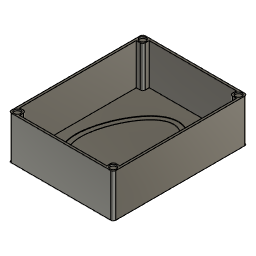
Wingspan - Eggs Container (Autodesk Fusion 360 design; units mm, degrees)
Autodesk Fusion 360 part; units mm, degrees
sketch "Skizze1" plane through (0, 0, 0) normal (0, 0, 1) x (1, 0, 0)
  line L0 (0, 0) -> (85, 0)
  line L1 (85, 0) -> (85, 109)
  line L2 (85, 109) -> (0, 109)
  line L3 (0, 109) -> (0, 0)
  dimension "d1" = 85
  dimension "d2" = 109
  constraint horizontal L0
  constraint vertical L1
  constraint horizontal L2
  constraint vertical L3
  constraint coincident L0.start L3.end
  measures "d1" distance of L0.start L0.end
  measures "d2" distance of L0.start L2.end
extrude "Extrusion16" add sketch "Skizze1" along normal blind 35
sketch "Skizze17" plane through (0, 0, 35) normal (0, 0, 1) x (-1, 0, 0)
  line L0 (0, -109) -> (0, 0)
  line L1 (0, 0) -> (-85, 0)
  line L2 (-85, 0) -> (-85, -109)
  line L3 (-85, -109) -> (0, -109)
  line L4 (0, -109) -> (-7, -109)
  line L5 (-7, -109) -> (-7, -102)
  line L6 (-7, -102) -> (0, -102)
  line L7 (0, -102) -> (0, -109)
  line L8 (-85, -109) -> (-78, -109)
  line L9 (-78, -109) -> (-78, -102)
  line L10 (-78, -102) -> (-85, -102)
  line L11 (-85, -102) -> (-85, -109)
  line L12 (0, 0) -> (-7, 0)
  line L13 (-7, 0) -> (-7, -7)
  line L14 (-7, -7) -> (0, -7)
  line L15 (0, -7) -> (0, 0)
  line L16 (-85, 0) -> (-78, 0)
  line L17 (-78, 0) -> (-78, -7)
  line L18 (-78, -7) -> (-85, -7)
  line L19 (-85, -7) -> (-85, 0)
  circle A0 centre (-3.5, -105.5) radius 2.65
  circle A1 centre (-81.5, -105.5) radius 2.65
  circle A2 centre (-81.5, -3.5) radius 2.65
  circle A3 centre (-3.5, -3.5) radius 2.65
  dimension "d148" = 7
  dimension "d149" = 7
  dimension "d150" = 7
  dimension "d151" = 7
  dimension "d152" = 7
  dimension "d153" = 7
  dimension "d154" = 7
  dimension "d155" = 7
  dimension "d156" = 5.3
  dimension "d157" = 5.3
  dimension "d158" = 5.3
  dimension "d159" = 5.3
  dimension "d160" = 3.5
  dimension "d161" = 3.5
  dimension "d162" = 3.5
  dimension "d163" = 3.5
  dimension "d164" = 3.5
  dimension "d165" = 3.5
  dimension "d166" = 3.5
  dimension "d167" = 3.5
  constraint horizontal L4
  constraint vertical L5
  constraint horizontal L6
  constraint vertical L7
  constraint coincident L0.start L3.end
  constraint horizontal L8
  constraint vertical L9
  constraint horizontal L10
  constraint vertical L11
  constraint coincident L2.end L3.start
  constraint horizontal L12
  constraint vertical L13
  constraint horizontal L14
  constraint vertical L15
  constraint coincident L0.end L1.start
  constraint horizontal L16
  constraint vertical L17
  constraint horizontal L18
  constraint vertical L19
  constraint coincident L1.end L2.start
  measures "d148" distance of L0.start L4.end
  measures "d149" distance of L0.start L6.end
  measures "d150" distance of L2.end L8.end
  measures "d151" distance of L2.end L10.end
  measures "d152" distance of L0.end L12.end
  measures "d153" distance of L0.end L14.end
  measures "d154" distance of L1.end L16.end
  measures "d155" distance of L1.end L18.end
  measures "d156" diameter of A0
  measures "d157" diameter of A1
  measures "d158" diameter of A2
  measures "d159" diameter of A3
  measures "d160" distance of L15 A3.centre
  measures "d161" distance of L14 A3.centre
  measures "d162" distance of L16 A2.centre
  measures "d163" distance of L19 A2.centre
  measures "d164" distance of L8 A1.centre
  measures "d165" distance of L11 A1.centre
  measures "d166" distance of L7 A0.centre
  measures "d167" distance of L4 A0.centre
sketch "Skizze18" plane through (0, 0, 35) normal (0, 0, 1) x (-1, 0, 0)
  line L0 (-78, -1.75) -> (-7, -1.75)
  line L1 (-7, -1.75) -> (-7, -107.25)
  line L2 (-7, -107.25) -> (-78, -107.25)
  line L3 (-78, -107.25) -> (-78, -1.75)
  line L4 (0, -109) -> (0, 0)
  line L5 (-78, 0) -> (-78, -7)
  line L6 (-85, 0) -> (-85, -109)
  line L7 (0, 0) -> (-85, 0)
  line L8 (-85, -109) -> (0, -109)
  dimension "d168" = 7
  dimension "d170" = 7
  dimension "d171" = 1.75
  dimension "d172" = 1.75
  constraint horizontal L0
  constraint vertical L1
  constraint horizontal L2
  constraint vertical L3
  measures "d168" distance of L1 L4
  measures "d170" distance of L3 L6
  measures "d171" distance of L0 L7
  measures "d172" distance of L2 L8
sketch "Skizze19" plane through (0, 0, 35) normal (0, 0, 1) x (-1, 0, 0)
  line L0 (-7, -7) -> (-1.75, -7)
  line L1 (-1.75, -7) -> (-1.75, -102)
  line L2 (-1.75, -102) -> (-7, -102)
  line L3 (-7, -102) -> (-7, -7)
  line L4 (0, 0) -> (-7, 0)
  line L5 (0, -109) -> (-7, -109)
  line L6 (0, -109) -> (0, 0)
  line L7 (-78, -7) -> (-83.25, -7)
  line L8 (-83.25, -7) -> (-83.25, -102)
  line L9 (-83.25, -102) -> (-78, -102)
  line L10 (-78, -102) -> (-78, -7)
  line L11 (-85, 0) -> (-85, -109)
  line L12 (-85, -109) -> (-78, -109)
  line L13 (-85, 0) -> (-78, 0)
  dimension "d174" = 7
  dimension "d175" = 7
  dimension "d176" = 7
  dimension "d177" = 1.75
  dimension "d178" = 1.75
  dimension "d179" = 7
  dimension "d180" = 7
  dimension "d181" = 7
  constraint horizontal L0
  constraint vertical L1
  constraint horizontal L2
  constraint vertical L3
  constraint horizontal L7
  constraint vertical L8
  constraint horizontal L9
  constraint vertical L10
  measures "d174" distance of L0 L4
  measures "d175" distance of L2 L5
  measures "d176" distance of L3 L6
  measures "d177" distance of L1 L6
  measures "d178" distance of L8 L11
  measures "d179" distance of L9 L12
  measures "d180" distance of L10 L11
  measures "d181" distance of L7 L13
extrude "Extrusion17" cut sketch "Skizze17" against normal blind 1.2 contours A0 | A1 | A2 | A3
extrude "Extrusion18" cut sketch "Skizze18" sketch "Skizze19" against normal blind 33.25 contours L0 L1 L2 L3 L5 of sketch 2
fillet "Abrundung5" radius 2 8 edges at (7, 102, 18.375) (78, 102, 18.375) (78, 7, 18.375) (7, 7, 18.375) (85, 109, 17.5) (0, 109, 17.5) (0, 0, 17.5) (85, 0, 17.5)
sketch "Skizze20" plane through (0, 0, 1.75) normal (0, 0, 1) x (-1, 0, 0)
  line L0 (-78, -104) -> (-78, -107.25)
  line L1 (-78, -107.25) -> (-7, -107.25)
  line L2 (-7, -107.25) -> (-7, -104)
  arc A0 (-5, -102) -> (-7, -104) centre (-5, -104) ccw
  line L3 (-5, -102) -> (-1.75, -102)
  line L4 (-1.75, -102) -> (-1.75, -7)
  line L5 (-1.75, -7) -> (-5, -7)
  arc A1 (-7, -5) -> (-5, -7) centre (-5, -5) ccw
  line L6 (-7, -5) -> (-7, -1.75)
  line L7 (-7, -1.75) -> (-78, -1.75)
  line L8 (-78, -1.75) -> (-78, -5)
  arc A2 (-80, -7) -> (-78, -5) centre (-80, -5) ccw
  line L9 (-80, -7) -> (-83.25, -7)
  line L10 (-83.25, -7) -> (-83.25, -102)
  line L11 (-83.25, -102) -> (-80, -102)
  arc A3 (-78, -104) -> (-80, -102) centre (-80, -104) ccw
  spline S0 degree 3 poles (-66.1211, -76.6115) (-59.4052, -88.6986) (-51.0157, -95.3555) (-42.4975, -95.3555) knots 0 0 0 0 1 1 1 1
  spline S1 degree 3 poles (-42.4975, -95.3555) (-33.9794, -95.3555) (-25.5902, -88.6986) (-18.874, -76.6115) knots 0 0 0 0 1 1 1 1
  spline S2 degree 3 poles (-18.874, -76.6115) (-13.324, -66.622) (-9.7378, -54.1768) (-9.7378, -44.9054) knots 0 0 0 0 1 1 1 1
  spline S3 degree 3 poles (-9.7378, -44.9054) (-9.7378, -35.9571) (-13.092, -27.5787) (-19.183, -21.3143) knots 0 0 0 0 1 1 1 1
  spline S4 degree 3 poles (-19.183, -21.3143) (-25.3273, -14.9941) (-33.6072, -11.5139) (-42.4979, -11.5139) knots 0 0 0 0 1 1 1 1
  spline S5 degree 3 poles (-42.4979, -11.5139) (-51.3886, -11.5139) (-59.6684, -14.9944) (-65.8128, -21.3143) knots 0 0 0 0 1 1 1 1
  spline S6 degree 3 poles (-65.8128, -21.3143) (-71.9035, -27.5791) (-75.2576, -35.9571) (-75.2576, -44.9054) knots 0 0 0 0 1 1 1 1
  spline S7 degree 3 poles (-75.2576, -44.9054) (-75.2573, -54.1768) (-71.671, -66.6223) (-66.1211, -76.6115) knots 0 0 0 0 1 1 1 1
  spline S8 degree 3 poles (-42.4975, -15.4416) (-26.3299, -15.4416) (-13.6658, -28.3836) (-13.6658, -44.9054) knots 0 0 0 0 1 1 1 1
  spline S9 degree 3 poles (-13.6658, -44.9054) (-13.6658, -62.4321) (-27.1411, -91.4275) (-42.4975, -91.4275) knots 0 0 0 0 1 1 1 1
  spline S10 degree 3 poles (-42.4975, -91.4275) (-57.854, -91.4275) (-71.3293, -62.4321) (-71.3293, -44.9054) knots 0 0 0 0 1 1 1 1
  spline S11 degree 3 poles (-71.3293, -44.9054) (-71.3293, -28.3836) (-58.6652, -15.4416) (-42.4975, -15.4416) knots 0 0 0 0 1 1 1 1
extrude "Extrusion19" cut sketch "Skizze20" against normal blind 0.4 contours S0 S1 S2 S3 S4 S5 S6 S7
extrude "Extrusion9" [suppressed]
sketch "Skizze14" plane through (0, 0, 35) normal (0, 0, 1) x (-1, 0, 0)
  line L0 (0, -115) -> (0, 0)
  line L1 (0, 0) -> (-85, 0)
  line L2 (-85, 0) -> (-85, -115)
  line L3 (-85, -115) -> (0, -115)
  line L4 (0, -115) -> (-7, -115)
  line L5 (-7, -115) -> (-7, -108)
  line L6 (-7, -108) -> (0, -108)
  line L7 (0, -108) -> (0, -115)
  line L8 (-85, -115) -> (-78, -115)
  line L9 (-78, -115) -> (-78, -108)
  line L10 (-78, -108) -> (-85, -108)
  line L11 (-85, -108) -> (-85, -115)
  line L12 (0, 0) -> (-7, 0)
  line L13 (-7, 0) -> (-7, -7)
  line L14 (-7, -7) -> (0, -7)
  line L15 (0, -7) -> (0, 0)
  line L16 (-85, 0) -> (-78, 0)
  line L17 (-78, 0) -> (-78, -7)
  line L18 (-78, -7) -> (-85, -7)
  line L19 (-85, -7) -> (-85, 0)
  circle A0 centre (-3.5, -111.5) radius 2.65
  circle A1 centre (-81.5, -111.5) radius 2.65
  circle A2 centre (-81.5, -3.5) radius 2.65
  circle A3 centre (-3.5, -3.5) radius 2.65
  dimension "d104" = 7
  dimension "d105" = 7
  dimension "d106" = 7
  dimension "d107" = 7
  dimension "d108" = 7
  dimension "d109" = 7
  dimension "d110" = 7
  dimension "d111" = 7
  dimension "d112" = 5.3
  dimension "d113" = 5.3
  dimension "d114" = 5.3
  dimension "d115" = 5.3
  dimension "d116" = 3.5
  dimension "d117" = 3.5
  dimension "d118" = 3.5
  dimension "d119" = 3.5
  dimension "d120" = 3.5
  dimension "d121" = 3.5
  dimension "d122" = 3.5
  dimension "d123" = 3.5
  constraint horizontal L4
  constraint vertical L5
  constraint horizontal L6
  constraint vertical L7
  constraint coincident L0.start L3.end
  constraint horizontal L8
  constraint vertical L9
  constraint horizontal L10
  constraint vertical L11
  constraint coincident L2.end L3.start
  constraint horizontal L12
  constraint vertical L13
  constraint horizontal L14
  constraint vertical L15
  constraint coincident L0.end L1.start
  constraint horizontal L16
  constraint vertical L17
  constraint horizontal L18
  constraint vertical L19
  constraint coincident L1.end L2.start
  measures "d104" distance of L0.start L4.end
  measures "d105" distance of L0.start L6.end
  measures "d106" distance of L2.end L8.end
  measures "d107" distance of L2.end L10.end
  measures "d108" distance of L0.end L12.end
  measures "d109" distance of L0.end L14.end
  measures "d110" distance of L1.end L16.end
  measures "d111" distance of L1.end L18.end
  measures "d112" diameter of A0
  measures "d113" diameter of A1
  measures "d114" diameter of A2
  measures "d115" diameter of A3
  measures "d116" distance of L15 A3.centre
  measures "d117" distance of L14 A3.centre
  measures "d118" distance of L19 A2.centre
  measures "d119" distance of L16 A2.centre
  measures "d120" distance of L11 A1.centre
  measures "d121" distance of L8 A1.centre
  measures "d122" distance of L5 A0.centre
  measures "d123" distance of L4 A0.centre
sketch "Skizze15" plane through (0, 0, 35) normal (0, 0, 1) x (-1, 0, 0)
  line L0 (-78, -113.25) -> (-7, -113.25)
  line L1 (-7, -113.25) -> (-7, -1.75)
  line L2 (-7, -1.75) -> (-78, -1.75)
  line L3 (-78, -1.75) -> (-78, -113.25)
  line L4 (0, 0) -> (-85, 0)
  line L5 (0, -115) -> (0, 0)
  line L6 (-85, -115) -> (0, -115)
  line L7 (-85, 0) -> (-85, -115)
  line L8 (-78, -108) -> (-83.25, -108)
  line L9 (-83.25, -108) -> (-83.25, -7)
  line L10 (-83.25, -7) -> (-78, -7)
  line L11 (-78, -7) -> (-78, -108)
  line L12 (-85, 0) -> (-78, 0)
  line L13 (-85, -115) -> (-78, -115)
  line L14 (-7, -108) -> (-1.75, -108)
  line L15 (-1.75, -108) -> (-1.75, -7)
  line L16 (-1.75, -7) -> (-7, -7)
  line L17 (-7, -7) -> (-7, -108)
  line L18 (-7, -7) -> (0, -7)
  line L19 (0, 0) -> (-7, 0)
  line L20 (0, -115) -> (-7, -115)
  dimension "d124" = 1.75
  dimension "d125" = 7
  dimension "d126" = 1.75
  dimension "d127" = 7
  dimension "d128" = 1.75
  dimension "d129" = 7
  dimension "d130" = 7
  dimension "d133" = 1.75
  dimension "d134" = 7
  dimension "d135" = 7
  constraint horizontal L0
  constraint vertical L1
  constraint horizontal L2
  constraint vertical L3
  constraint horizontal L8
  constraint vertical L9
  constraint horizontal L10
  constraint vertical L11
  constraint coincident L3 L8.start
  constraint horizontal L14
  constraint vertical L15
  constraint horizontal L16
  constraint vertical L17
  constraint coincident L1 L14.start
  measures "d124" distance of L2 L4
  measures "d125" distance of L1 L5
  measures "d126" distance of L0 L6
  measures "d127" distance of L3 L7
  measures "d128" distance of L7 L9
  measures "d129" distance of L10 L12
  measures "d130" distance of L8 L13
  measures "d133" distance of L5 L15
  measures "d134" distance of L14 L20
  measures "d135" distance of L16 L19
extrude "Extrusion13" [suppressed]
extrude "Extrusion14" [suppressed]
sketch "Skizze16" plane through (0, 0, 1.75) normal (0, 0, 1) x (-1, 0, 0)
  line L0 (-7, -1.75) -> (-78, -1.75)
  line L1 (-78, -1.75) -> (-78, -7)
  line L2 (-78, -7) -> (-83.25, -7)
  line L3 (-83.25, -7) -> (-83.25, -108)
  line L4 (-83.25, -108) -> (-78, -108)
  line L5 (-78, -108) -> (-78, -113.25)
  line L6 (-78, -113.25) -> (-7, -113.25)
  line L7 (-7, -113.25) -> (-7, -108)
  line L8 (-7, -108) -> (-1.75, -108)
  line L9 (-1.75, -108) -> (-1.75, -7)
  line L10 (-1.75, -7) -> (-7, -7)
  line L11 (-7, -7) -> (-7, -1.75)
  spline S0 degree 3 poles (-64.8008, -78.3152) (-58.6523, -89.381) (-50.9717, -95.4755) (-43.1733, -95.4755) knots 0 0 0 0 1 1 1 1
  spline S1 degree 3 poles (-43.1733, -95.4755) (-35.3749, -95.4755) (-27.6945, -89.381) (-21.5458, -78.3152) knots 0 0 0 0 1 1 1 1
  spline S2 degree 3 poles (-21.5458, -78.3152) (-16.4648, -69.1698) (-13.1816, -57.7762) (-13.1816, -49.2882) knots 0 0 0 0 1 1 1 1
  spline S3 degree 3 poles (-13.1816, -49.2882) (-13.1816, -41.096) (-16.2524, -33.4256) (-21.8287, -27.6904) knots 0 0 0 0 1 1 1 1
  spline S4 degree 3 poles (-21.8287, -27.6904) (-27.4539, -21.9043) (-35.0341, -18.7182) (-43.1736, -18.7182) knots 0 0 0 0 1 1 1 1
  spline S5 degree 3 poles (-43.1736, -18.7182) (-51.313, -18.7182) (-58.8933, -21.9046) (-64.5185, -27.6904) knots 0 0 0 0 1 1 1 1
  spline S6 degree 3 poles (-64.5185, -27.6904) (-70.0945, -33.4259) (-73.1653, -41.096) (-73.1653, -49.2882) knots 0 0 0 0 1 1 1 1
  spline S7 degree 3 poles (-73.1653, -49.2882) (-73.165, -57.7762) (-69.8817, -69.1701) (-64.8008, -78.3152) knots 0 0 0 0 1 1 1 1
  spline S8 degree 3 poles (-43.1733, -22.3139) (-28.3718, -22.3139) (-16.7777, -34.1625) (-16.7777, -49.2882) knots 0 0 0 0 1 1 1 1
  spline S9 degree 3 poles (-16.7777, -49.2882) (-16.7777, -65.334) (-29.1144, -91.8794) (-43.1733, -91.8794) knots 0 0 0 0 1 1 1 1
  spline S10 degree 3 poles (-43.1733, -91.8794) (-57.2322, -91.8794) (-69.5689, -65.334) (-69.5689, -49.2882) knots 0 0 0 0 1 1 1 1
  spline S11 degree 3 poles (-69.5689, -49.2882) (-69.5689, -34.1625) (-57.9748, -22.3139) (-43.1733, -22.3139) knots 0 0 0 0 1 1 1 1
extrude "Extrusion15" [suppressed]
fillet "Abrundung3" [suppressed]
fillet "Abrundung4" [suppressed]
sketch "Skizze11" plane through (0, 0, 35) normal (0, 0, 1) x (-1, 0, 0)
  line L0 (0, -115) -> (0, 0)
  line L1 (0, 0) -> (-85, 0)
  line L2 (-85, 0) -> (-85, -115)
  line L3 (-85, -115) -> (0, -115)
  line L4 (0, -115) -> (-7, -115)
  line L5 (-7, -115) -> (-7, -108)
  line L6 (-7, -108) -> (0, -108)
  line L7 (0, -108) -> (0, -115)
  line L8 (-85, -115) -> (-78, -115)
  line L9 (-78, -115) -> (-78, -108)
  line L10 (-78, -108) -> (-85, -108)
  line L11 (-85, -108) -> (-85, -115)
  line L12 (0, 0) -> (-7, 0)
  line L13 (-7, 0) -> (-7, -7)
  line L14 (-7, -7) -> (0, -7)
  line L15 (0, -7) -> (0, 0)
  line L16 (-85, 0) -> (-78, 0)
  line L17 (-78, 0) -> (-78, -7)
  line L18 (-78, -7) -> (-85, -7)
  line L19 (-85, -7) -> (-85, 0)
  circle A0 centre (-3.5, -3.5) radius 2.65
  circle A1 centre (-81.5, -3.5) radius 2.65
  circle A2 centre (-3.5, -111.5) radius 2.65
  circle A3 centre (-81.5, -111.5) radius 2.65
  dimension "d65" = 7
  dimension "d66" = 7
  dimension "d67" = 7
  dimension "d68" = 7
  dimension "d69" = 7
  dimension "d70" = 7
  dimension "d71" = 7
  dimension "d72" = 7
  dimension "d73" = 5.3
  dimension "d74" = 5.3
  dimension "d75" = 5.3
  dimension "d76" = 5.3
  dimension "d77" = 3.5
  dimension "d78" = 3.5
  dimension "d79" = 3.5
  dimension "d80" = 3.5
  dimension "d81" = 3.5
  dimension "d82" = 3.5
  dimension "d83" = 3.5
  dimension "d84" = 3.5
  constraint horizontal L4
  constraint vertical L5
  constraint horizontal L6
  constraint vertical L7
  constraint coincident L0.start L3.end
  constraint horizontal L8
  constraint vertical L9
  constraint horizontal L10
  constraint vertical L11
  constraint coincident L2.end L3.start
  constraint horizontal L12
  constraint vertical L13
  constraint horizontal L14
  constraint vertical L15
  constraint coincident L0.end L1.start
  constraint horizontal L16
  constraint vertical L17
  constraint horizontal L18
  constraint vertical L19
  constraint coincident L1.end L2.start
  measures "d65" distance of L0.start L4.end
  measures "d66" distance of L0.start L6.end
  measures "d67" distance of L2.end L8.end
  measures "d68" distance of L2.end L10.end
  measures "d69" distance of L0.end L12.end
  measures "d70" distance of L0.end L14.end
  measures "d71" distance of L1.end L16.end
  measures "d72" distance of L1.end L18.end
  measures "d73" diameter of A0
  measures "d74" diameter of A1
  measures "d75" diameter of A2
  measures "d76" diameter of A3
  measures "d77" distance of L12 A0.centre
  measures "d78" distance of L13 A0.centre
  measures "d79" distance of L16 A1.centre
  measures "d80" distance of L19 A1.centre
  measures "d81" distance of L11 A3.centre
  measures "d82" distance of L10 A3.centre
  measures "d83" distance of L6 A2.centre
  measures "d84" distance of L5 A2.centre
sketch "Skizze12" plane through (0, 0, 35) normal (0, 0, 1) x (-1, 0, 0)
  line L0 (-78, -1.75) -> (-7, -1.75)
  line L1 (-7, -1.75) -> (-7, -113.25)
  line L2 (-7, -113.25) -> (-78, -113.25)
  line L3 (-78, -113.25) -> (-78, -1.75)
  line L4 (-85, -115) -> (0, -115)
  line L5 (0, 0) -> (-85, 0)
  line L6 (0, -115) -> (0, 0)
  line L7 (-85, 0) -> (-85, -115)
  line L8 (-78, -7) -> (-83.25, -7)
  line L9 (-83.25, -7) -> (-83.25, -108)
  line L10 (-83.25, -108) -> (-78, -108)
  line L11 (-78, -108) -> (-78, -7)
  line L12 (-85, -115) -> (-78, -115)
  line L13 (-85, 0) -> (-78, 0)
  line L14 (-7, -7.2335) -> (-1.75, -7.2335)
  line L15 (-1.75, -7.2335) -> (-1.75, -108)
  line L16 (-1.75, -108) -> (-7, -108)
  line L17 (-7, -108) -> (-7, -7.2335)
  line L18 (-7, -108) -> (0, -108)
  line L19 (0, -115) -> (-7, -115)
  dimension "d85" = 1.75
  dimension "d86" = 1.75
  dimension "d87" = 7
  dimension "d88" = 7
  dimension "d89" = 7
  dimension "d90" = 7
  dimension "d91" = 1.75
  dimension "d92" = 1.75
  dimension "d93" = 7
  constraint horizontal L0
  constraint vertical L1
  constraint horizontal L2
  constraint vertical L3
  constraint horizontal L8
  constraint vertical L9
  constraint horizontal L10
  constraint vertical L11
  constraint coincident L3 L8.start
  constraint horizontal L14
  constraint vertical L15
  constraint horizontal L16
  constraint vertical L17
  constraint coincident L1 L14.start
  measures "d85" distance of L2 L4
  measures "d86" distance of L0 L5
  measures "d87" distance of L1 L6
  measures "d88" distance of L3 L7
  measures "d89" distance of L10 L12
  measures "d90" distance of L8 L13
  measures "d91" distance of L7 L9
  measures "d92" distance of L6 L15
  measures "d93" distance of L18 L19
extrude "Extrusion10" [suppressed]
extrude "Extrusion11" [suppressed]
sketch "Skizze13" plane through (0, 0, 6.75) normal (0, 0, 1) x (-1, 0, 0)
  line L0 (-7, -113.25) -> (-7, -108)
  line L1 (-7, -108) -> (-1.75, -108)
  line L2 (-1.75, -108) -> (-1.75, -7.2335)
  line L3 (-1.75, -7.2335) -> (-7, -7.2335)
  line L4 (-7, -7.2335) -> (-7, -1.75)
  line L5 (-7, -1.75) -> (-78, -1.75)
  line L6 (-78, -1.75) -> (-78, -7)
  line L7 (-78, -7) -> (-83.25, -7)
  line L8 (-83.25, -7) -> (-83.25, -108)
  line L9 (-83.25, -108) -> (-78, -108)
  line L10 (-78, -108) -> (-78, -113.25)
  line L11 (-78, -113.25) -> (-7, -113.25)
  spline S0 degree 3 poles (-61.8748, -78.6389) (-56.1896, -88.8708) (-49.0877, -94.5061) (-41.8769, -94.5061) knots 0 0 0 0 1 1 1 1
  spline S1 degree 3 poles (-41.8769, -94.5061) (-34.6661, -94.5061) (-27.5645, -88.8708) (-21.8791, -78.6389) knots 0 0 0 0 1 1 1 1
  spline S2 degree 3 poles (-21.8791, -78.6389) (-17.1809, -70.1825) (-14.1451, -59.6474) (-14.1451, -51.799) knots 0 0 0 0 1 1 1 1
  spline S3 degree 3 poles (-14.1451, -51.799) (-14.1451, -44.2241) (-16.9845, -37.1316) (-22.1406, -31.8286) knots 0 0 0 0 1 1 1 1
  spline S4 degree 3 poles (-22.1406, -31.8286) (-27.342, -26.4785) (-34.3511, -23.5325) (-41.8772, -23.5325) knots 0 0 0 0 1 1 1 1
  spline S5 degree 3 poles (-41.8772, -23.5325) (-49.4033, -23.5325) (-56.4124, -26.4788) (-61.6137, -31.8286) knots 0 0 0 0 1 1 1 1
  spline S6 degree 3 poles (-61.6137, -31.8286) (-66.7696, -37.1319) (-69.609, -44.2241) (-69.609, -51.799) knots 0 0 0 0 1 1 1 1
  spline S7 degree 3 poles (-69.609, -51.799) (-69.6087, -59.6474) (-66.5729, -70.1828) (-61.8748, -78.6389) knots 0 0 0 0 1 1 1 1
  spline S8 degree 3 poles (-41.8769, -26.8573) (-28.1907, -26.8573) (-17.4702, -37.813) (-17.4702, -51.799) knots 0 0 0 0 1 1 1 1
  spline S9 degree 3 poles (-17.4702, -51.799) (-17.4702, -66.6357) (-28.8773, -91.181) (-41.8769, -91.181) knots 0 0 0 0 1 1 1 1
  spline S10 degree 3 poles (-41.8769, -91.181) (-54.8765, -91.181) (-66.2836, -66.6357) (-66.2836, -51.799) knots 0 0 0 0 1 1 1 1
  spline S11 degree 3 poles (-66.2836, -51.799) (-66.2836, -37.813) (-55.5631, -26.8573) (-41.8769, -26.8573) knots 0 0 0 0 1 1 1 1
extrude "Extrusion12" [suppressed]
fillet "Abrundung1" [suppressed]
fillet "Abrundung2" [suppressed]
extrude "Extrusion1" [suppressed]
sketch "Skizze2" plane through (0, 0, 30) normal (0, 0, 1) x (-1, 0, 0)
  line L0 (0, -115) -> (0, 0)
  line L1 (0, 0) -> (-85, 0)
  line L2 (-85, 0) -> (-85, -115)
  line L3 (-85, -115) -> (0, -115)
  line L4 (0, -115) -> (-7, -115)
  line L5 (-7, -115) -> (-7, -108)
  line L6 (-7, -108) -> (0, -108)
  line L7 (0, -108) -> (0, -115)
  line L8 (-85, -115) -> (-78, -115)
  line L9 (-78, -115) -> (-78, -108)
  line L10 (-78, -108) -> (-85, -108)
  line L11 (-85, -108) -> (-85, -115)
  line L12 (-85, 0) -> (-78, 0)
  line L13 (-78, 0) -> (-78, -7)
  line L14 (-78, -7) -> (-85, -7)
  line L15 (-85, -7) -> (-85, 0)
  line L16 (0, 0) -> (-7, 0)
  line L17 (-7, 0) -> (-7, -7)
  line L18 (-7, -7) -> (0, -7)
  line L19 (0, -7) -> (0, 0)
  circle A0 centre (-3.5, -3.5) radius 2.65
  circle A1 centre (-81.5, -3.5) radius 2.65
  circle A2 centre (-81.5, -111.5) radius 2.65
  circle A3 centre (-3.5, -111.5) radius 2.65
  dimension "d5" = 7
  dimension "d6" = 7
  dimension "d7" = 7
  dimension "d8" = 7
  dimension "d9" = 7
  dimension "d10" = 7
  dimension "d11" = 7
  dimension "d12" = 7
  dimension "d13" = 5.3
  dimension "d14" = 5.3
  dimension "d15" = 5.3
  dimension "d16" = 5.3
  dimension "d17" = 3.5
  dimension "d18" = 3.5
  dimension "d19" = 3.5
  dimension "d20" = 3.5
  dimension "d21" = 3.5
  dimension "d22" = 3.5
  dimension "d23" = 3.5
  dimension "d24" = 3.5
  constraint horizontal L4
  constraint vertical L5
  constraint horizontal L6
  constraint vertical L7
  constraint coincident L0.start L3.end
  constraint horizontal L8
  constraint vertical L9
  constraint horizontal L10
  constraint vertical L11
  constraint coincident L2.end L3.start
  constraint horizontal L12
  constraint vertical L13
  constraint horizontal L14
  constraint vertical L15
  constraint coincident L1.end L2.start
  constraint horizontal L16
  constraint vertical L17
  constraint horizontal L18
  constraint vertical L19
  constraint coincident L0.end L1.start
  measures "d5" distance of L0.start L4.end
  measures "d6" distance of L0.start L6.end
  measures "d7" distance of L2.end L8.end
  measures "d8" distance of L2.end L10.end
  measures "d9" distance of L1.end L12.end
  measures "d10" distance of L1.end L14.end
  measures "d11" distance of L0.end L16.end
  measures "d12" distance of L0.end L18.end
  measures "d13" diameter of A0
  measures "d14" diameter of A1
  measures "d15" diameter of A2
  measures "d16" diameter of A3
  measures "d17" distance of L7 A3.centre
  measures "d18" distance of L4 A3.centre
  measures "d19" distance of L10 A2.centre
  measures "d20" distance of L11 A2.centre
  measures "d21" distance of L15 A1.centre
  measures "d22" distance of L14 A1.centre
  measures "d23" distance of L16 A0.centre
  measures "d24" distance of L17 A0.centre
sketch "Skizze3" plane through (0, 0, 30) normal (0, 0, 1) x (-1, 0, 0)
  line L0 (-78, -1.75) -> (-7, -1.75)
  line L1 (-7, -1.75) -> (-7, -113.25)
  line L2 (-7, -113.25) -> (-78, -113.25)
  line L3 (-78, -113.25) -> (-78, -1.75)
  line L4 (0, 0) -> (-85, 0)
  line L5 (-85, -115) -> (0, -115)
  line L6 (-78, -115) -> (-78, -108)
  line L7 (-85, 0) -> (-85, -115)
  line L8 (0, -115) -> (0, 0)
  dimension "d25" = 1.75
  dimension "d26" = 1.75
  dimension "d28" = 7
  dimension "d29" = 7
  constraint horizontal L0
  constraint vertical L1
  constraint horizontal L2
  constraint vertical L3
  measures "d25" distance of L0 L4
  measures "d26" distance of L2 L5
  measures "d28" distance of L3 L7
  measures "d29" distance of L1 L8
extrude "Extrusion2" [suppressed]
sketch "Skizze5" plane through (0, 0, 30) normal (0, 0, 1) x (-1, 0, 0)
  line L0 (-78, -1.75) -> (-7, -1.75)
  line L1 (-7, -1.75) -> (-7, -113.25)
  line L2 (-7, -113.25) -> (-78, -113.25)
  line L3 (-78, -113.25) -> (-78, -1.75)
  line L4 (0, -115) -> (0, 0)
  line L5 (0, 0) -> (-85, 0)
  line L6 (-85, 0) -> (-85, -115)
  line L7 (-85, -115) -> (0, -115)
  line L8 (-7, -108) -> (-1.75, -108)
  line L9 (-1.75, -108) -> (-1.75, -22)
  line L10 (-1.75, -22) -> (-7, -22)
  line L11 (-7, -22) -> (-7, -108)
  line L12 (0, -115) -> (0, 0)
  line L13 (0, -115) -> (-7, -115)
  dimension "d33" = 1.75
  dimension "d34" = 86
  dimension "d35" = 7
  constraint horizontal L8
  constraint vertical L9
  constraint horizontal L10
  constraint vertical L11
  constraint coincident L1 L8.start
  measures "d33" distance of L9 L12
  measures "d34" distance of L8 L10
  measures "d35" distance of L8 L13
sketch "Skizze6" plane through (0, 0, 30) normal (0, 0, 1) x (-1, 0, 0)
  line L0 (-7, -7) -> (-1.75, -7)
  line L1 (-1.75, -7) -> (-1.75, -93)
  line L2 (-1.75, -93) -> (-7, -93)
  line L3 (-7, -93) -> (-7, -7)
  line L4 (0, -115) -> (0, 0)
  line L5 (0, 0) -> (-7, 0)
  line L6 (-78, -22) -> (-83.25, -22)
  line L7 (-83.25, -22) -> (-83.25, -108)
  line L8 (-83.25, -108) -> (-78, -108)
  line L9 (-78, -108) -> (-78, -22)
  line L10 (-85, 0) -> (-85, -115)
  line L11 (-85, -115) -> (-78, -115)
  line L12 (-78, -7) -> (-85, -7)
  line L13 (-85, 0) -> (-78, 0)
  dimension "d36" = 86
  dimension "d37" = 1.75
  dimension "d38" = 7
  dimension "d39" = 7
  dimension "d44" = 1.75
  dimension "d45" = 7
  dimension "d47" = 86
  dimension "d48" = 7
  constraint horizontal L0
  constraint vertical L1
  constraint horizontal L2
  constraint vertical L3
  constraint horizontal L6
  constraint vertical L7
  constraint horizontal L8
  constraint vertical L9
  measures "d36" distance of L0 L2
  measures "d37" distance of L1 L4
  measures "d38" distance of L0 L5
  measures "d39" distance of L3 L4
  measures "d44" distance of L7 L10
  measures "d45" distance of L8 L11
  measures "d47" distance of L6 L8
  measures "d48" distance of L9 L10
extrude "Extrusion3" [suppressed]
extrude "Extrusion4" [suppressed]
extrude "Extrusion5" [suppressed]
sketch "Skizze7" plane through (0, 0, 1.75) normal (0, 0, 1) x (-1, 0, 0)
  line L0 (-7, -7) -> (-7, -1.75)
  line L1 (-7, -1.75) -> (-78, -1.75)
  line L2 (-78, -1.75) -> (-78, -22)
  line L3 (-78, -22) -> (-83.25, -22)
  line L4 (-83.25, -22) -> (-83.25, -108)
  line L5 (-83.25, -108) -> (-78, -108)
  line L6 (-78, -108) -> (-78, -113.25)
  line L7 (-78, -113.25) -> (-7, -113.25)
  line L8 (-7, -113.25) -> (-7, -93)
  line L9 (-7, -93) -> (-1.75, -93)
  line L10 (-1.75, -93) -> (-1.75, -7)
  line L11 (-1.75, -7) -> (-7, -7)
  spline S0 degree 3 poles (-57.2282, -66.5179) (-52.2019, -75.5641) (-45.9231, -80.5463) (-39.5479, -80.5463) knots 0 0 0 0 1 1 1 1
  spline S1 degree 3 poles (-39.5479, -80.5463) (-33.1727, -80.5463) (-26.8941, -75.5641) (-21.8675, -66.5179) knots 0 0 0 0 1 1 1 1
  spline S2 degree 3 poles (-21.8675, -66.5179) (-17.7139, -59.0415) (-15.0298, -49.7273) (-15.0298, -42.7885) knots 0 0 0 0 1 1 1 1
  spline S3 degree 3 poles (-15.0298, -42.7885) (-15.0298, -36.0914) (-17.5402, -29.8208) (-22.0988, -25.1324) knots 0 0 0 0 1 1 1 1
  spline S4 degree 3 poles (-22.0988, -25.1324) (-26.6973, -20.4022) (-32.8942, -17.7976) (-39.5481, -17.7976) knots 0 0 0 0 1 1 1 1
  spline S5 degree 3 poles (-39.5481, -17.7976) (-46.2021, -17.7976) (-52.3989, -20.4025) (-56.9975, -25.1324) knots 0 0 0 0 1 1 1 1
  spline S6 degree 3 poles (-56.9975, -25.1324) (-61.5558, -29.8211) (-64.0662, -36.0914) (-64.0662, -42.7885) knots 0 0 0 0 1 1 1 1
  spline S7 degree 3 poles (-64.0662, -42.7885) (-64.0659, -49.7273) (-61.3819, -59.0418) (-57.2282, -66.5179) knots 0 0 0 0 1 1 1 1
  spline S8 degree 3 poles (-39.5479, -20.7371) (-27.4477, -20.7371) (-17.9696, -30.4232) (-17.9696, -42.7885) knots 0 0 0 0 1 1 1 1
  spline S9 degree 3 poles (-17.9696, -42.7885) (-17.9696, -55.9058) (-28.0548, -77.6065) (-39.5479, -77.6065) knots 0 0 0 0 1 1 1 1
  spline S10 degree 3 poles (-39.5479, -77.6065) (-51.041, -77.6065) (-61.1261, -55.9058) (-61.1261, -42.7885) knots 0 0 0 0 1 1 1 1
  spline S11 degree 3 poles (-61.1261, -42.7885) (-61.1262, -30.4232) (-51.648, -20.7371) (-39.5479, -20.7371) knots 0 0 0 0 1 1 1 1
sketch "Skizze9" plane through (0, 0, 30) normal (0, 0, 1) x (-1, 0, 0)
  line L0 (-83.25, -22) -> (-78, -22)
  line L1 (-78, -22) -> (-78, -1.75)
  line L2 (-78, -1.75) -> (-7, -1.75)
  line L3 (-7, -1.75) -> (-7, -7)
  line L4 (-7, -7) -> (-1.75, -7)
  line L5 (-1.75, -7) -> (-1.75, -93)
  line L6 (-1.75, -93) -> (-7, -93)
  line L7 (-7, -93) -> (-7, -113.25)
  line L8 (-7, -113.25) -> (-78, -113.25)
  line L9 (-78, -113.25) -> (-78, -108)
  line L10 (-78, -108) -> (-83.25, -108)
  line L11 (-83.25, -108) -> (-83.25, -22)
  circle A0 centre (-81.5, -3.5) radius 2.65
  circle A1 centre (-81.5, -111.5) radius 2.65
  circle A2 centre (-3.5, -3.5) radius 2.65
  circle A3 centre (-3.5, -111.5) radius 2.65
  line L12 (0, -115) -> (0, 0)
  line L13 (0, 0) -> (-85, 0)
  line L14 (-85, 0) -> (-85, -115)
  line L15 (-85, -115) -> (0, -115)
  line L16 (-7, -93) -> (-1.75, -93)
  line L17 (-1.75, -93) -> (-1.75, -108)
  line L18 (-1.75, -108) -> (-7, -108)
  line L19 (-7, -108) -> (-7, -93)
  line L20 (-78, -22) -> (-83.25, -22)
  line L21 (-83.25, -22) -> (-83.25, -7)
  line L22 (-83.25, -7) -> (-78, -7)
  line L23 (-78, -7) -> (-78, -22)
  dimension "d55" = 1.75
  dimension "d56" = 7
  dimension "d57" = 1.75
  dimension "d58" = 7
  constraint horizontal L16
  constraint vertical L17
  constraint horizontal L18
  constraint vertical L19
  constraint coincident L6.end L7.start
  constraint horizontal L20
  constraint vertical L21
  constraint horizontal L22
  constraint vertical L23
  constraint coincident L0.end L1.start
  measures "d55" distance of L12 L17
  measures "d56" distance of L15 L18
  measures "d57" distance of L14 L21
  measures "d58" distance of L13 L22
extrude "Extrusion7" [suppressed]
sketch "Skizze10" plane through (0, 0, 1.75) normal (0, 0, 1) x (-1, 0, 0)
  line L0 (-7, -7) -> (-7, -1.75)
  line L1 (-7, -1.75) -> (-78, -1.75)
  line L2 (-78, -1.75) -> (-78, -7)
  line L3 (-78, -7) -> (-83.25, -7)
  line L4 (-83.25, -7) -> (-83.25, -108)
  line L5 (-83.25, -108) -> (-78, -108)
  line L6 (-78, -108) -> (-78, -113.25)
  line L7 (-78, -113.25) -> (-7, -113.25)
  line L8 (-7, -113.25) -> (-7, -108)
  line L9 (-7, -108) -> (-1.75, -108)
  line L10 (-1.75, -108) -> (-1.75, -7)
  line L11 (-1.75, -7) -> (-7, -7)
  spline S0 degree 3 poles (-64.8028, -78.627) (-58.4872, -89.9936) (-50.5977, -96.2538) (-42.5872, -96.2538) knots 0 0 0 0 1 1 1 1
  spline S1 degree 3 poles (-42.5872, -96.2538) (-34.5767, -96.2538) (-26.6876, -89.9936) (-20.3717, -78.627) knots 0 0 0 0 1 1 1 1
  spline S2 degree 3 poles (-20.3717, -78.627) (-15.1525, -69.2328) (-11.78, -57.5294) (-11.78, -48.8107) knots 0 0 0 0 1 1 1 1
  spline S3 degree 3 poles (-11.78, -48.8107) (-11.78, -40.3957) (-14.9343, -32.5167) (-20.6623, -26.6256) knots 0 0 0 0 1 1 1 1
  spline S4 degree 3 poles (-20.6623, -26.6256) (-26.4404, -20.6822) (-34.2268, -17.4094) (-42.5875, -17.4094) knots 0 0 0 0 1 1 1 1
  spline S5 degree 3 poles (-42.5875, -17.4094) (-50.9483, -17.4094) (-58.7346, -20.6825) (-64.5128, -26.6256) knots 0 0 0 0 1 1 1 1
  spline S6 degree 3 poles (-64.5128, -26.6256) (-70.2404, -32.517) (-73.3947, -40.3957) (-73.3947, -48.8107) knots 0 0 0 0 1 1 1 1
  spline S7 degree 3 poles (-73.3947, -48.8107) (-73.3944, -57.5294) (-70.0219, -69.2331) (-64.8028, -78.627) knots 0 0 0 0 1 1 1 1
  spline S8 degree 3 poles (-42.5872, -21.103) (-27.3832, -21.103) (-15.4739, -33.2736) (-15.4739, -48.8107) knots 0 0 0 0 1 1 1 1
  spline S9 degree 3 poles (-15.4739, -48.8107) (-15.4739, -65.2927) (-28.146, -92.5599) (-42.5872, -92.5599) knots 0 0 0 0 1 1 1 1
  spline S10 degree 3 poles (-42.5872, -92.5599) (-57.0284, -92.5599) (-69.7005, -65.2927) (-69.7005, -48.8107) knots 0 0 0 0 1 1 1 1
  spline S11 degree 3 poles (-69.7005, -48.8107) (-69.7005, -33.2736) (-57.7912, -21.103) (-42.5872, -21.103) knots 0 0 0 0 1 1 1 1
extrude "Extrusion8" [suppressed]
extrude "Extrusion6" [suppressed]
sketch "Skizze8" plane through (0, 0, 30) normal (0, 0, 1) x (-1, 0, 0)
  line L0 (-78, -7) -> (-78, -1.75)
  line L1 (-78, -1.75) -> (-7, -1.75)
  line L2 (-7, -1.75) -> (-7, -7)
  line L3 (-7, -7) -> (-1.75, -7)
  line L4 (-1.75, -7) -> (-1.75, -108)
  line L5 (-7, -113.25) -> (-78, -113.25)
  line L6 (-78, -113.25) -> (-78, -108)
  line L7 (-78, -108) -> (-83.25, -108)
  line L8 (-83.25, -108) -> (-83.25, -7)
  circle A0 centre (-81.5, -3.5) radius 2.65
  circle A1 centre (-81.5, -111.5) radius 2.65
  circle A2 centre (-3.5, -3.5) radius 2.65
  circle A3 centre (-3.5, -111.5) radius 2.65
  line L9 (0, -115) -> (0, 0)
  line L10 (0, 0) -> (-85, 0)
  line L11 (-85, 0) -> (-85, -115)
  line L12 (-85, -115) -> (0, -115)
  line L13 (-7, -93) -> (-2, -93)
  line L14 (-2, -93) -> (-2, -108)
  line L15 (-2, -108) -> (-7, -108)
  line L16 (-7, -108) -> (-7, -93)
  line L17 (-83.25, -7) -> (-78, -7)
  line L18 (-1.75, -108) -> (-7, -108)
  line L19 (-7, -108) -> (-7, -113.25)
  dimension "d53" = 5
  dimension "d54" = 15
  constraint horizontal L13
  constraint vertical L14
  constraint horizontal L15
  constraint vertical L16
  measures "d53" distance of L13.start L13.end
  measures "d54" distance of L13.start L15.end
equation "d31 = -30 mm + 1.75 mm"
equation "d34 = 100 mm - 14 mm"
equation "d42 = -30 mm + 1.75 mm"
equation "d49 = -30 mm + 1.75 mm"
equation "d59 = -30 mm + 1.75 mm"
equation "d94 = -30 mm + 1.75 mm"
equation "d136 = -35 mm + 1.75 mm"
equation "d184 = -35 mm + 1.75 mm"
